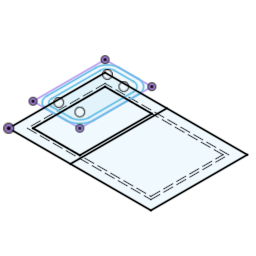
Assignment 5 - CNC_UPDATE v4 (Autodesk Fusion 360 design; units mm, degrees)
Autodesk Fusion 360 part; units mm, degrees
note: some values were not read from the file. Chosen so that the rebuilt part matches the saved one: which bodies a step acts on. Set by a fixed rule: which sketch regions a step uses.
sketch "Sketch1" plane through (0, 0, 0) normal (0, 0, 1) x (1, 0, 0)
  line L0 (0, 0) -> (152, 0)
  line L1 (152, 0) -> (152, 103)
  line L2 (152, 103) -> (0, 103)
  line L3 (0, 103) -> (0, 0)
  line L4 (10, 10) -> (142, 10) construction
  line L5 (142, 10) -> (142, 93) construction
  line L6 (142, 93) -> (10, 93) construction
  line L7 (10, 93) -> (10, 10) construction
  line L8 (139, 13) -> (139, 90) construction
  line L9 (139, 90) -> (13, 90) construction
  line L10 (13, 90) -> (13, 13) construction
  line L11 (13, 13) -> (139, 13) construction
  line L12 (13, 13) -> (63, 13)
  line L13 (63, 13) -> (63, 90)
  line L14 (63, 90) -> (13, 90)
  line L15 (13, 90) -> (13, 13)
  line L16 (66, 0) -> (66, 103)
  dimension "d3" = 152
  dimension "d4" = 103
  dimension "d11" = -13
  dimension "d12" = 50
  dimension "d15" = 3
  constraint horizontal L0
  constraint vertical L1
  constraint horizontal L2
  constraint vertical L3
  constraint coincident L0.start L3.end
  constraint horizontal L12
  constraint vertical L13
  constraint horizontal L14
  constraint vertical L15
  constraint coincident L2 L16.end
  constraint coincident L0 L16.start
  measures "d3" distance of L0.start L0.end
  measures "d4" distance of L0.start L2.end
  measures "d12" distance of L10.end L12.end
extrude "Extrude1" add sketch "Sketch1" against normal blind 12.5 contours L0 L2 L3 L16 | L0 L1 L2 L16 | L12 L13 L14 L15 makes body 1
extrude "Extrude2" add sketch "Sketch1" along normal blind 25 separate body contours L0 L2 L3 L16 | L0 L1 L2 L16 | L12 L13 L14 L15 makes body 2
extrude "Extrude3" add sketch "Sketch1" along normal blind 25 separate body contours L12 L13 L14 L15 makes body 3
fillet "Fillet1" radius 12.5 8 edges at (38, 13, 25) (13, 51.5, 25) (38, 90, 25) (63, 51.5, 25) (13, 13, 12.5) (63, 13, 12.5) (13, 90, 12.5) (63, 90, 12.5) on bodies 3
extrude "Extrude4" add sketch "Sketch1" along normal blind 25 separate body contours L12 L13 L14 L15 makes body 4
sketch "Sketch2" plane through (0, 0, 25) normal (0, 0, 1) x (-1, 0, 0)
  line L0 (-13, -90) -> (-13, -13)
  line L1 (-13, -13) -> (-63, -13)
  line L2 (-63, -13) -> (-63, -90)
  line L3 (-63, -90) -> (-13, -90)
  line L4 (-48, -13) -> (-28, -13)
  line L5 (-15.5, -25.5) -> (-15.5, -77.5)
  line L6 (-28, -90) -> (-48, -90)
  line L7 (-63, -75) -> (-63, -28)
  arc A0 (-48, -13) -> (-63, -28) centre (-48, -28) ccw
  arc A1 (-15.5, -25.5) -> (-28, -13) centre (-28, -25.5) ccw
  arc A2 (-63, -75) -> (-48, -90) centre (-48, -75) ccw
  arc A3 (-28, -90) -> (-15.5, -77.5) centre (-28, -77.5) ccw
  line L8 (-48, -18) -> (-28, -18)
  arc A4 (-20.5, -25.5) -> (-28, -18) centre (-28, -25.5) ccw
  line L9 (-20.5, -25.5) -> (-20.5, -77.5)
  arc A5 (-28, -85) -> (-20.5, -77.5) centre (-28, -77.5) ccw
  line L10 (-28, -85) -> (-48, -85)
  arc A6 (-58, -75) -> (-48, -85) centre (-48, -75) ccw
  line L11 (-58, -75) -> (-58, -28)
  arc A7 (-48, -18) -> (-58, -28) centre (-48, -28) ccw
  dimension "d25" = 15
  dimension "d26" = 12.5
  dimension "d27" = 15
  dimension "d28" = 12.5
  constraint horizontal L4
  constraint vertical L5
  constraint horizontal L6
  constraint vertical L7
  constraint tangent L7 A0
  constraint tangent L4 A0
  constraint tangent L4 A1
  constraint tangent L5 A1
  constraint tangent L6 A2
  constraint tangent L7 A2
  constraint tangent L5 A3
  constraint tangent L6 A3
  measures "d25" radius of A0
  measures "d26" radius of A1
  measures "d27" radius of A2
  measures "d28" radius of A3
extrude "Extrude5" cut sketch "Sketch2" against normal blind 20 contours L8 A4 L9 A5 L10 A6 L11 A7 bodies 4
fillet "Fillet2" radius 5 8 edges at (22.6967, 20.1967, 5) (20.5, 51.5, 5) (22.6967, 82.8033, 5) (38, 85, 5) (55.0711, 82.0711, 5) (58, 51.5, 5) (55.0711, 20.9289, 5) (38, 18, 5) on bodies 4
copy_body "CopyPasteBodies1" bodies 2 makes body 5
combine "Combine1" operation cut target body 5 tool bodies 4 keep tools makes body 6 at (122.3333, 64.3333, 0)
combine "Combine2" operation add target body 6 tool bodies 4 keep tools
copy_body "CopyPasteBodies2" bodies 1 makes body 7
copy_body "CopyPasteBodies3" bodies 7 makes body 8
copy_body "CopyPasteBodies4" bodies 6 makes body 9
copy_body "CopyPasteBodies5" bodies 3 makes body 10
combine "Combine3" operation add target body 9 tool bodies 7
extrude "Extrude6" add sketch "Sketch1" along normal blind 25 contours L0 L1 L2 L16 bodies 8
combine "Combine4" operation add target body 10 tool bodies 8
extrude "Extrude7" add 1 faces at (4.3333, 42.8333, 0) along direction (0, 0, 1) blind 2 on bodies 10 bodies 10
extrude "Extrude8" cut 1 faces at (66, 34.3333, 9.6667) along direction (1, 0, 0) blind 10 on bodies 10 bodies 10
extrude "Extrude9" add sketch "Sketch2" against normal blind 12.55 separate body contours L0 L1 L3 L5 A1 A3 | L1 L2 L3 L4 L5 L6 L7 A0 A1 A2 A3 | L2 L3 A2 | L1 L2 A0 | L8 A4 L9 A5 L10 A6 L11 A7 makes body 11
extrude "Extrude10" add 1 faces at (4.3333, 60.1667, 2) along direction (0, 0, 1) up to surface (10.45 mm away) separate body on bodies 10 makes body 12
combine "Combine5" operation add target body 10 tool bodies 12
hidden bodies 4 5 9 10 11
equation "Width = 103 mm"
equation "length = 152 mm"
equation "d3 = length"
equation "d4 = Width"
equation "SafetyOffset = 10 mm"
equation "d6 = -SafetyOffset"
equation "mdf = 12.5 mm"
equation "ABS = 25 mm"
equation "W2 = 3 in"
equation "D1 = 50 mm"
equation "d12 = D1"
equation "d13 = -mdf"
equation "d16 = ABS"
equation "d18 = ABS"
equation "B_FILLET = 12.5 mm"
equation "d22 = B_FILLET"
equation "d23 = ABS"
equation "d26 = B_FILLET"
equation "d28 = B_FILLET"
equation "Wall = 5 mm"
equation "d30 = -Wall"
equation "Inset = ABS - Wall"
equation "d32 = -Inset"
equation "d35 = Wall"
equation "d36 = ABS"
equation "FlipTab = 2 mm"
equation "d39 = FlipTab"
equation "F_CollisionOffset = 10 mm"
equation "d42 = -F_CollisionOffset"
named bodies: "MDF BASE", "ABS_GENERIC", "ObjectFlip", "ABS_GENERIC (1)", "Object_Top", "MDF BASE (1)", "MDF BASE (1) (1)", "Bowl_FirstCut", "Bowl_Second Cut"
